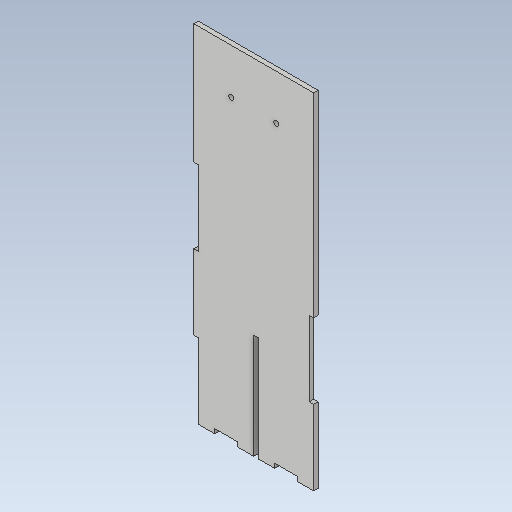
# Autodesk Inventor part: Pared Garita3
Saved by Autodesk Inventor 2020 (Build 240168000, 168)
## iProperties
Created: 2020-03-09
Part Number: Pared Garita3
Material: Genérico
Document SubType Name: Modeling
Designer: Diego Guillén
Density: 1 g/cm^3
Appearance: Valor por defecto
Author: Diego Guillén
Autodesk Inventor part; units mm, degrees
ref_plane "YZ Plane" through (0, 0, 0) normal (1, 0, 0) x (0, 1, 0)
ref_plane "XZ Plane" through (0, 0, 0) normal (0, 1, 0) x (-1, 0, 0)
ref_plane "XY Plane" through (0, 0, 0) normal (0, 0, 1) x (1, 0, 0)
sketch "Boceto1" plane through (0, 0, 0) normal (0, 0, 1) x (1, 0, 0)
  line L0 (0, 0) -> (80, 0)
  line L1 (80, 0) -> (80, 230)
  line L2 (80, 230) -> (0, 230)
  line L3 (0, 230) -> (0, 0)
  dimension "d0" = 80
  dimension "d1" = 230
  constraints: 8 end point, 2 parallel, 1 horizontal, 1 perpendicular
  measures "d0" distance of L1.end L2.end
  measures "d1" distance of L0.end L1.end
extrude "Extrusión1" add sketch "Boceto1" along normal blind 3
sketch "Boceto2" plane through (0, 0, 3) normal (0, 0, 1) x (1, 0, 0)
  line L0 (0, 0) -> (80, 0) construction
  line L1 (80, 0) -> (80, 230) construction
  line L2 (80, 230) -> (0, 230) construction
  line L3 (0, 230) -> (0, 0) construction
  line L4 (3, 0) -> (0, 0)
  line L5 (0, 0) -> (0, 50)
  line L6 (0, 50) -> (3, 50)
  line L7 (3, 50) -> (3, 0)
  line L8 (0, 230) -> (17.5445, 230)
  line L9 (77, 100) -> (80, 100)
  line L10 (80, 100) -> (80, 50)
  line L11 (80, 50) -> (77, 50)
  line L12 (77, 50) -> (77, 100)
  line L13 (80, 0) -> (80, 230) construction
  line L14 (0, 150) -> (3, 150)
  line L15 (3, 150) -> (3, 100)
  line L16 (3, 100) -> (0, 100)
  line L17 (0, 100) -> (0, 150)
  line L18 (0, 230) -> (0, 0) construction
  point P0 (80, 115)
  dimension "d4" = 3
  dimension "d5" = 50
  dimension "d8" = 50
  dimension "d9" = 3
  dimension "d16" = 50
  dimension "d17" = 3
  dimension "d18" = 50
  dimension "d19" = 50
  constraints: 26 end point, 6 parallel, 4 horizontal, 3 perpendicular, 2 collinear, 1 coincident, 1 midpoint
  measures "d4" distance of L5.end L6.end
  measures "d5" distance of L6.end L4.start
  measures "d8" distance of L11.end L9.start
  measures "d9" distance of L10.end L11.end
  measures "d16" distance between parallel lines of L0 L11
  measures "d17" distance of L15.end L16.end
  measures "d18" distance of L14.end L15.end
  measures "d19" distance between parallel lines of L16 L6
extrude "Extrusión2" cut sketch "Boceto2" against normal blind 3
sketch "Boceto3" plane through (0, 0, 3) normal (0, 0, 1) x (1, 0, 0)
  line L0 (3, 50) -> (3, 0) construction
  line L1 (3, 0) -> (80, 0) construction
  line L2 (80, 0) -> (80, 50) construction
  line L3 (80, 50) -> (77, 50) construction
  line L4 (77, 50) -> (77, 100) construction
  line L5 (77, 100) -> (80, 100) construction
  line L6 (80, 100) -> (80, 230) construction
  line L7 (80, 230) -> (0, 230) construction
  line L8 (0, 230) -> (0, 150) construction
  line L9 (0, 50) -> (3, 50) construction
  line L10 (40, 70) -> (43, 70)
  line L11 (43, 70) -> (43, 0)
  line L12 (43, 0) -> (40, 0)
  line L13 (40, 0) -> (40, 70)
  line L14 (3, 0) -> (80, 0) construction
  line L15 (0, 150) -> (3, 150) projected
  line L16 (3, 150) -> (3, 100) projected
  line L17 (3, 100) -> (0, 100) projected
  line L18 (0, 100) -> (0, 50) projected
  point P0 (0, 0)
  point P1 (41.5, 0)
  point P2 (41.5, 0)
  dimension "d12" = 3
  dimension "d13" = 70
  constraints: 8 end point, 2 midpoint, 2 parallel, 1 coincident, 1 collinear, 1 horizontal, 1 perpendicular
  measures "d12" distance of L11.end L12.end
  measures "d13" distance of L12.end L10.start
extrude "Extrusión3" cut sketch "Boceto3" against normal blind 10
sketch "Boceto4" plane through (0, 0, 3) normal (0, 0, 1) x (1, 0, 0)
  line L0 (43, 70) -> (43, 0) construction
  line L1 (43, 0) -> (80, 0) construction
  line L2 (80, 0) -> (80, 50) construction
  line L3 (80, 50) -> (77, 50) construction
  line L4 (77, 50) -> (77, 100) construction
  line L5 (77, 100) -> (80, 100) construction
  line L6 (80, 100) -> (80, 230) construction
  line L7 (80, 230) -> (0, 230) construction
  line L8 (0, 230) -> (0, 150) construction
  line L9 (0, 150) -> (3, 150) construction
  line L10 (3, 150) -> (3, 100) construction
  line L11 (3, 100) -> (0, 100) construction
  line L12 (0, 100) -> (0, 50) construction
  line L13 (0, 50) -> (3, 50) construction
  line L14 (3, 50) -> (3, 0) construction
  line L15 (3, 0) -> (40, 0) construction
  line L16 (40, 0) -> (40, 70) construction
  line L17 (40, 70) -> (43, 70) construction
  point P0 (0, 0)
  point P1 (25, 200)
  point P2 (55, 200)
  dimension "d20" = 30
  dimension "d21" = 30
  dimension "d23" = 25
  dimension "d24" = 30
  measures "d20" distance from line of L7 point (25, 200)
  measures "d21" distance from line of L7 point (55, 200)
  measures "d23" distance from line of L8 point (25, 200)
  measures "d24" distance of point (55, 200) point (25, 200)
hole "Agujero1" at (25, 200, 3) at (55, 200, 3) direction (0, 0, -1) diameter 3.3 end through all both
sketch "Boceto5" plane through (0, 0, 3) normal (0, 0, 1) x (1, 0, 0)
  circle A0 centre (25, 200) radius 1.65 construction
  circle A1 centre (55, 200) radius 1.65 construction
  line L0 (43, 70) -> (43, 0) construction
  line L1 (43, 0) -> (80, 0) construction
  line L2 (80, 0) -> (80, 50) construction
  line L3 (80, 50) -> (77, 50) construction
  line L4 (77, 50) -> (77, 100) construction
  line L5 (77, 100) -> (80, 100) construction
  line L6 (80, 100) -> (80, 230) construction
  line L7 (80, 230) -> (0, 230) construction
  line L8 (0, 230) -> (0, 150) construction
  line L9 (0, 150) -> (3, 150) construction
  line L10 (3, 150) -> (3, 100) construction
  line L11 (3, 100) -> (0, 100) construction
  line L12 (0, 100) -> (0, 50) construction
  line L13 (0, 50) -> (3, 50) construction
  line L14 (3, 50) -> (3, 0) construction
  line L15 (3, 0) -> (40, 0) construction
  line L16 (40, 0) -> (40, 70) construction
  line L17 (40, 70) -> (43, 70) construction
  line L18 (14, 3) -> (29, 3)
  line L19 (29, 3) -> (29, 0)
  line L20 (29, 0) -> (14, 0)
  line L21 (14, 0) -> (14, 3)
  line L22 (54, 3) -> (69, 3)
  line L23 (69, 3) -> (69, 0)
  line L24 (69, 0) -> (54, 0)
  line L25 (54, 0) -> (54, 3)
  line L26 (3, 0) -> (40, 0) construction
  line L27 (43, 0) -> (80, 0) construction
  point P0 (0, 0)
  point P1 (21.5, 0)
  point P2 (21.5, 0)
  point P3 (61.5, 0)
  point P4 (61.5, 0)
  dimension "d32" = 3
  dimension "d33" = 3
  dimension "d35" = 15
  dimension "d36" = 15
  constraints: 16 end point, 4 midpoint, 4 parallel, 2 coincident, 2 collinear, 2 horizontal, 2 perpendicular
  measures "d32" distance of L18.end L19.end
  measures "d33" distance of L22.end L23.end
  measures "d35" distance of L18.start L18.end
  measures "d36" distance of L22.start L22.end
extrude "Extrusión4" cut sketch "Boceto5" against normal blind 10
equation "\"d8\" = d7"
equation "\"d9\" = d4"
equation "\"d21\" = d20"
equation "\"d7\" = d5"
